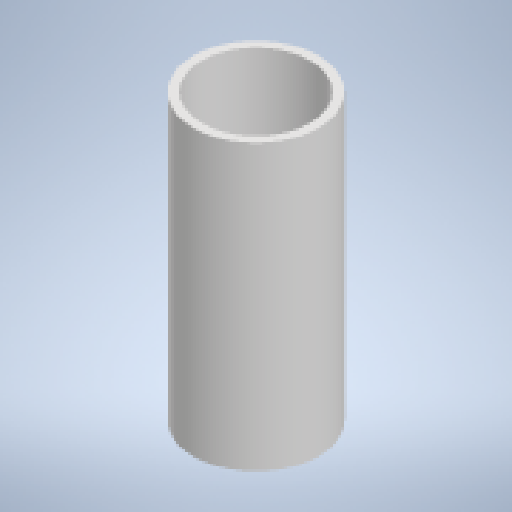
# Autodesk Inventor part: pvc 3 in tube
Saved by Autodesk Inventor 2025 (Build 290162010, 162A)
## iProperties
Created: 2024-06-12
Part Number: pvc 3 in tube
Material: Generic
Document SubType Name: Modeling
Designer: ngensadmin
Density: 1 g/cm^3
Appearance: Default
Author: ngensadmin
Autodesk Inventor part; units mm, degrees
ref_plane "YZ Plane" through (0, 0, 0) normal (1, 0, 0) x (0, 1, 0)
ref_plane "XZ Plane" through (0, 0, 0) normal (0, 1, 0) x (-1, 0, 0)
ref_plane "XY Plane" through (0, 0, 0) normal (0, 0, 1) x (1, 0, 0)
sketch "Sketch1" plane through (0, 0, 0) normal (0, 1, 0) x (-1, 0, 0)
  circle A0 centre (0, 0) radius 44.8
  circle A1 centre (0, 0) radius 38.65
  dimension "d0" = 89.6
  dimension "d1" = 77.3
  constraints: 2 centre point, 2 coincident
  measures "d0" diameter of A0
  measures "d1" diameter of A1
extrude "Extrusion1" add sketch "Sketch1" along normal blind 203.2
body "Solid1"
